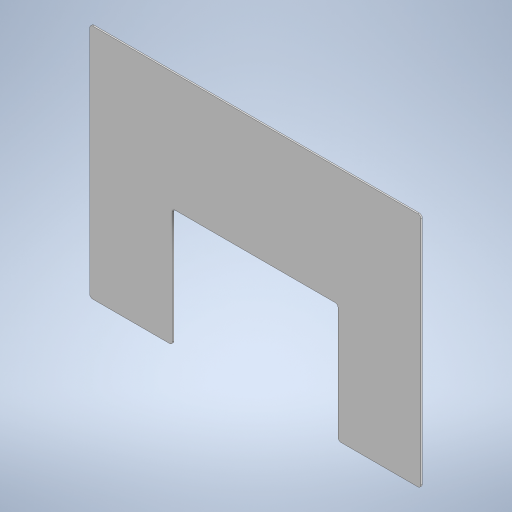
# Autodesk Inventor part: Blocker
Saved by Autodesk Inventor 2023 (Build 270158000, 158)
## iProperties
Created: 2023-10-25
Part Number: Blocker
Material: Generic
Document SubType Name: Modeling
Designer: Robodox
Density: 1 g/cm^3
Appearance: Default
Author: Robodox
Autodesk Inventor part; units mm, degrees
ref_plane "YZ Plane" through (0, 0, 0) normal (1, 0, 0) x (0, 1, 0)
ref_plane "XZ Plane" through (0, 0, 0) normal (0, 1, 0) x (-1, 0, 0)
ref_plane "XY Plane" through (0, 0, 0) normal (0, 0, 1) x (1, 0, 0)
sketch "Sketch1" plane through (0, 0, 0) normal (0, 0, 1) x (1, 0, 0)
  line L0 (-177.8, 127) -> (177.8, 127)
  line L1 (177.8, 127) -> (177.8, -127)
  line L2 (177.8, -127) -> (-177.8, -127)
  line L3 (-177.8, -127) -> (-177.8, 127)
  line L4 (-88.8998, 127) -> (-88.8998, -127)
  line L5 (88.9077, 127) -> (88.9077, -127)
  line L6 (-88.8998, 0) -> (88.9077, 0)
  point P0 (0, 0)
  dimension "d0" = 355.6
  dimension "d1" = 254
  constraints: 14 end point, 4 point on line, 3 perpendicular, 2 midpoint, 2 parallel, 1 horizontal
  measures "d0" distance of L0.start L0.end
  measures "d1" distance of L2.end L0.start
extrude "Extrusion1" add sketch "Sketch1" along normal blind 1.5875 contours L0 L4 L2 L3 | L0 L5 L6 L4 | L0 L1 L2 L5
fillet "Fillet1" radius 3.175 1 edges at (177.8, 127, 0.7937)
fillet "Fillet2" radius 3.175 1 edges at (177.8, -127, 0.7937)
fillet "Fillet3" radius 3.175 1 edges at (-88.8998, -127, 0.7937)
fillet "Fillet4" radius 3.175 1 edges at (-88.8998, 0, 0.7937)
fillet "Fillet5" radius 3.175 1 edges at (-177.8, -127, 0.7937)
fillet "Fillet6" radius 3.175 1 edges at (-177.8, 127, 0.7937)
fillet "Fillet7" radius 3.175 1 edges at (88.9077, -127, 0.7937)
fillet "Fillet8" radius 3.175 1 edges at (88.9077, 0, 0.7937)
body "Solid1"
